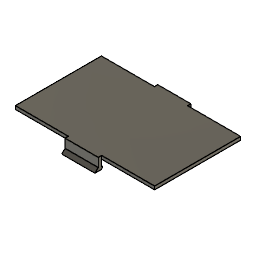
ensamble brazo (Autodesk Fusion 360 archive; units mm, degrees)
design "Tapa Pilas"
part number: 2026-08-17-13-49-44-268
Autodesk Fusion 360 part; units mm, degrees
sketch "Boceto1" plane through (0, 0, 0) normal (0, 0, 1) x (1, 0, 0)
  line L0 (41.9, 25.9) -> (-41.9, 25.9)
  line L1 (-41.9, 25.9) -> (-41.9, -25.9)
  line L2 (-41.9, -25.9) -> (41.9, -25.9)
  line L3 (41.9, -25.9) -> (41.9, 25.9)
  line L4 (41.9, 25.9) -> (-41.9, -25.9) construction
  line L5 (-41.9, 25.9) -> (41.9, -25.9) construction
  dimension "d1" = 83.8
  dimension "d2" = 51.8
  constraint horizontal L0
  constraint perpendicular L0 L1
  constraint parallel L0 L2
  constraint parallel L1 L3
  constraint coincident L4 origin
  constraint coincident L5 origin
  measures "d1" distance of L1.end L2.end
  measures "d2" distance of L0.end L1.end
extrude "Extruir1" add sketch "Boceto1" along normal blind 2
sketch "Boceto4" plane through (0, 0, 0) normal (1, 0, 0) x (0, 1, 0)
  line L0 (25.9, 2) -> (27.9, 2)
  line L1 (27.9, 2) -> (27.9, -5.3)
  line L2 (27.9, -5.3) -> (25.9, -5.3)
  line L3 (25.9, -5.3) -> (25.9, 2)
  line L4 (25.9, -5.3) -> (24.8996, -3.8)
  line L5 (25.9, -5.3) -> (27.703, -5.3) construction
  line L6 (24.8996, -3.8) -> (25.9, -3.8)
  line L7 (27.9, -5.3) -> (29.9, -5.3)
  line L8 (27.9, -5.3) -> (27.9, -3.3)
  line L9 (27.9, -3.3) -> (29.9, -5.3)
  line L10 (0, 7.5) -> (0, -4)
  line L11 (-25.9, -5.3) -> (-25.9, 2)
  line L12 (-25.9, 2) -> (-27.9, 2)
  line L13 (-27.9, 2) -> (-27.9, -5.3)
  line L14 (-27.9, -5.3) -> (-29.9, -5.3)
  line L15 (-27.9, -5.3) -> (-27.9, -3.3)
  line L16 (-27.9, -3.3) -> (-29.9, -5.3)
  line L17 (-24.8996, -3.8) -> (-25.9, -3.8)
  line L18 (-25.9, -5.3) -> (-24.8996, -3.8)
  line L19 (-25.9, -5.3) -> (-27.703, -5.3) construction
  line L20 (-27.9, -5.3) -> (-25.9, -5.3)
  dimension "d20" = 2
  dimension "d21" = 7.3
  dimension "d29" = 1.0004
  dimension "d30" = 1.803
  dimension "d31" = 2
  dimension "d32" = 2
  constraint horizontal L0
  constraint vertical L1
  constraint horizontal L2
  constraint vertical L3
  constraint horizontal L5
  constraint coincident L3 L6.end
  constraint perpendicular L3 L6
  constraint perpendicular L1 L7
  constraint perpendicular L7 L8
  constraint vertical L10
  constraint symmetric L0.start L10 L11.end
  constraint symmetric L0.end L10 L12.end
  constraint symmetric L1.end L10 L13.end
  constraint symmetric L2.end L10 L11.start
  constraint symmetric L4.end L10 L17.start
  constraint symmetric L5.end L10 L19.end
  constraint symmetric L6.end L10 L17.end
  constraint symmetric L7.end L10 L14.end
  constraint symmetric L8.end L10 L15.end
  measures "d20" distance of L0.start L0.end
  measures "d21" distance of L0.start L2.end
  measures "d29" distance of L4.end L6.end
  measures "d30" distance of L2.end L4.end
  measures "d31" distance of L1.end L7.end
  measures "d32" distance of L1.end L8.end
extrude "Extruir5" add sketch "Boceto4" along normal mid plane 20
fillet "Empalme1" radius 0.25 2 edges at (0, 24.8996, -3.8) (0, -24.8996, -3.8)
equation "d21 = 2 mm + 5.3 mm"
equation "d15 = 84.6 mm - 79.8 mm"
equation "d17 = ( ( 48.6 / 2 ) * 1 mm ) - 3.6 mm"

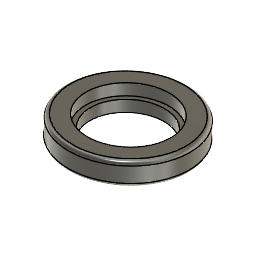
design "seguro clip"
part number: 2026-06-24-11-01-33-015
Autodesk Fusion 360 part; units mm, degrees
sketch "Boceto1" plane through (0, 0, 0) normal (1, 0, 0) x (0, 1, 0)
  circle A0 centre (0, 0) radius 8
  circle A1 centre (0, 0) radius 4.9
  dimension "d1" = 16
  dimension "d2" = 9.8
  constraint coincident A0.centre A1.centre
  measures "d1" diameter of A0
  measures "d2" diameter of A1
extrude "Extruir1" add sketch "Boceto1" against normal blind 3
move_body "Desplazar1" bodies 1 to x (0, -0.036999, -0.999315) y (0.732785, 0.679994, -0.025177) z (0.68046, -0.732283, 0.027113) at (0, 0, 0)
fillet "Empalme1" radius 0.5 1 faces at (5.2911, 6.0332, 0.7773)
sketch "Boceto3" plane through (0, 0.111, 2.9979) normal (0, 0.036999, 0.999315) x (-1, 0, 0)
  circle A0 centre (0, 0) radius 4.9
  circle A1 centre (0, 0) radius 7.5
  circle A2 centre (0, 0) radius 5.5
  dimension "d10" = 11
  constraint concentric A0 A2
  measures "d10" diameter of A2
extrude "Extruir3" cut sketch "Boceto3" against normal blind 1.5 contours A0 | A2
